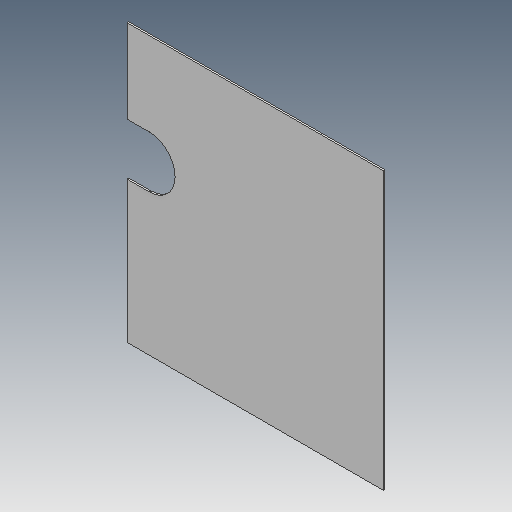
# Autodesk Inventor part: Part78
Saved by Autodesk Inventor 2020.5 (Build 245400000, 400)
## iProperties
Created: 2022-11-26
Part Number: Part78
Material: 一般
Document SubType Name: Modeling
Designer: Administrator
Density: 1 g/cm^3
Appearance: 既定
Author: Administrator
Autodesk Inventor part; units mm, degrees
ref_plane "YZ Plane" through (0, 0, 0) normal (1, 0, 0) x (0, 1, 0)
ref_plane "XZ Plane" through (0, 0, 0) normal (0, 1, 0) x (-1, 0, 0)
ref_plane "XY Plane" through (0, 0, 0) normal (0, 0, 1) x (1, 0, 0)
sketch "スケッチ1" plane through (0, 0, 0) normal (0, 0, 1) x (1, 0, 0)
  circle A0 centre (-15.5, 0) radius 2.5 projected
  circle A1 centre (15.5, 0) radius 2.5 projected
  circle A2 centre (0, 0) radius 11 projected
  line L0 (-15.1987, 13) -> (15.1987, 13) projected
  arc A3 (15.1987, -13) -> (15.1987, 13) centre (0, 0) ccw projected
  line L1 (15.1987, -13) -> (-15.1987, -13) projected
  arc A4 (-15.1987, 13) -> (-15.1987, -13) centre (0, 0) ccw projected
  circle A5 centre (-15.5, -130.182) radius 2.5 projected
  circle A6 centre (15.5, -130.182) radius 2.5 projected
  circle A7 centre (0, -130.182) radius 11 projected
  line L2 (-15.1987, -143.182) -> (15.1987, -143.182) projected
  arc A8 (-15.1987, -117.182) -> (-15.1987, -143.182) centre (0, -130.182) ccw projected
  line L3 (15.1987, -117.182) -> (-15.1987, -117.182) projected
  arc A9 (15.1987, -143.182) -> (15.1987, -117.182) centre (0, -130.182) ccw projected
  circle A10 centre (0, -130.182) radius 5 projected
  circle A11 centre (0, 0) radius 5 projected
  line L4 (-29, -33.3408) -> (-29, 14.909) projected
  line L5 (119, -145.0901) -> (-29, -145.0901) projected
  line L6 (-29, -63.3408) -> (-29, -33.3408)
  line L7 (119, 16.9081) -> (119, 16.909) projected
  line L8 (119, -145.0901) -> (119, 14.909)
  line L9 (119, 14.909) -> (119, 14.909)
  line L10 (119, 14.909) -> (119, -145.0901)
  line L11 (119, -145.0901) -> (119, -145.0901)
  circle A12 centre (0, -130.1819) radius 55
  circle A13 centre (0, 0.0009) radius 55
  line L12 (119, -145.0901) -> (59, -145.0901)
  line L13 (59, -145.0901) -> (59, 14.909)
  line L14 (59, 14.909) -> (119, 14.909)
  line L15 (119, 14.909) -> (119, -145.0901)
  line L16 (119, 14.909) -> (-29, 14.909) projected
  line L17 (119, 14.909) -> (119, -145.0901) projected
  line L18 (-16.25, -33.3408) -> (-29, -33.3408) projected
  line L19 (-29, -145.0901) -> (-29, -63.3408) projected
  line L20 (-29, -63.3408) -> (-16.25, -63.3408) projected
  arc A14 (-16.25, -63.3408) -> (-16.25, -33.3408) centre (-16.25, -48.3408) ccw projected
  circle A15 centre (-15.5, -130.1819) radius 3 projected
  circle A16 centre (-15.5, 0.0009) radius 3 projected
  circle A17 centre (69, -105.0901) radius 2 projected
  line L21 (99, -5.091) -> (80, -5.091) projected
  line L22 (80, -5.091) -> (80, -55.091) projected
  line L23 (80, -55.091) -> (99, -55.091) projected
  line L24 (99, -55.091) -> (99, -5.091) projected
  circle A18 centre (69, -65.0901) radius 2 projected
  circle A19 centre (0, 0.0009) radius 6 projected
  circle A20 centre (0, -130.1819) radius 6 projected
  circle A21 centre (15.5, -130.1819) radius 3 projected
  circle A22 centre (89, 4.909) radius 2 projected
  circle A23 centre (89, -135.0901) radius 1.5 projected
  line L25 (80, -125.0901) -> (99, -125.0901) projected
  line L26 (99, -125.0901) -> (99, -75.0901) projected
  line L27 (99, -75.0901) -> (80, -75.0901) projected
  line L28 (80, -75.0901) -> (80, -125.0901) projected
  circle A24 centre (69, -25.0901) radius 2 projected
  circle A25 centre (15.5, 0.0009) radius 3 projected
  circle A26 centre (14.75, -81.8408) radius 15 projected
  point P0 (0, 0)
  dimension "d2" = 110
  dimension "d3" = 110
  dimension "d4" = 60
  dimension "d5" = 159.9991
  constraints: 18 end point, 4 equal length, 2 centre point, 2 perpendicular, 1 point on line, 1 vertical
  measures "d2" diameter of A12
  measures "d3" diameter of A13
  measures "d4" distance of L10.end L12.end
  measures "d5" distance between parallel lines of L14 L12
extrude "押し出し1" add sketch "スケッチ1" along normal blind 1 contours A0 | A1 | A2 | L0 A3 L1 A4 | A5 | A6 | A7 | A8 L3 A9 L2 | A10 | A11 | L4 L16 A13 A14 L18 | L16 L13 L5 A12 A26 L19 L20 A14 A13 | L14 L8 L5 L13 | A12 A26 L5 L19 | A26 A12 | A12 A26 | A15 | A16 | A17 | L24 L23 L22 L21 | A18 | A19 | A20 | A21 | A22 | A23 | L28 L27 L26 L25 | A24 | A25
